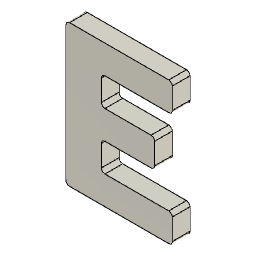
East (Autodesk Fusion 360 design; units mm, degrees)
Autodesk Fusion 360 part; units mm, degrees
sketch "Sketch1" plane through (0, 0, 0) normal (0, 1, 0) x (1, 0, 0)
  line L0 (0, -1.27) -> (0, -49.53)
  line L1 (1.27, -50.8) -> (36.83, -50.8)
  line L2 (38.1, -49.53) -> (38.1, -41.91)
  line L3 (36.83, -40.64) -> (13.97, -40.64)
  line L4 (12.7, -39.37) -> (12.7, -31.75)
  line L5 (13.97, -30.48) -> (30.4855, -30.48)
  line L6 (31.7555, -29.21) -> (31.7555, -21.59)
  line L7 (30.4855, -20.32) -> (13.97, -20.32)
  line L8 (12.7, -19.05) -> (12.7, -11.43)
  line L9 (13.97, -10.16) -> (36.83, -10.16)
  line L10 (38.1, -8.89) -> (38.1, -1.27)
  line L11 (36.83, 0) -> (1.27, 0)
  arc A0 (0, -49.53) -> (1.27, -50.8) centre (1.27, -49.53) ccw
  arc A1 (36.83, -50.8) -> (38.1, -49.53) centre (36.83, -49.53) ccw
  arc A2 (38.1, -41.91) -> (36.83, -40.64) centre (36.83, -41.91) ccw
  arc A3 (12.7, -39.37) -> (13.97, -40.64) centre (13.97, -39.37) ccw
  arc A4 (13.97, -30.48) -> (12.7, -31.75) centre (13.97, -31.75) ccw
  arc A5 (30.4855, -30.48) -> (31.7555, -29.21) centre (30.4855, -29.21) ccw
  arc A6 (31.7555, -21.59) -> (30.4855, -20.32) centre (30.4855, -21.59) ccw
  arc A7 (12.7, -19.05) -> (13.97, -20.32) centre (13.97, -19.05) ccw
  arc A8 (13.97, -10.16) -> (12.7, -11.43) centre (13.97, -11.43) ccw
  arc A9 (36.83, -10.16) -> (38.1, -8.89) centre (36.83, -8.89) ccw
  arc A10 (38.1, -1.27) -> (36.83, 0) centre (36.83, -1.27) ccw
  arc A11 (1.27, 0) -> (0, -1.27) centre (1.27, -1.27) ccw
  point P0 (0, -50.8)
  dimension "d1" = 50.8
  dimension "d2" = 1.27
  constraint vertical L0
  constraint perpendicular L0 L1
  constraint perpendicular L1 L2
  constraint perpendicular L2 L3
  constraint perpendicular L3 L4
  constraint perpendicular L4 L5
  constraint perpendicular L5 L6
  constraint perpendicular L6 L7
  constraint perpendicular L7 L8
  constraint perpendicular L8 L9
  constraint perpendicular L9 L10
  constraint perpendicular L0 L11
  constraint coincident P0 L0
  constraint coincident P0 L1
  constraint tangent L0 A0
  constraint tangent L1 A0
  constraint tangent L1 A1
  constraint tangent L2 A1
  constraint equal A0 A1
  constraint tangent L2 A2
  constraint tangent L3 A2
  constraint equal A0 A2
  constraint tangent L3 A3
  constraint tangent L4 A3
  constraint equal A0 A3
  constraint tangent L4 A4
  constraint tangent L5 A4
  constraint equal A0 A4
  constraint tangent L5 A5
  constraint tangent L6 A5
  constraint equal A0 A5
  constraint tangent L6 A6
  constraint tangent L7 A6
  constraint equal A0 A6
  constraint tangent L7 A7
  constraint tangent L8 A7
  constraint equal A0 A7
  constraint tangent L8 A8
  constraint tangent L9 A8
  constraint equal A0 A8
  constraint tangent L9 A9
  constraint tangent L10 A9
  constraint equal A0 A9
  constraint tangent L10 A10
  constraint tangent L11 A10
  constraint equal A0 A10
  constraint coincident origin L0
  constraint tangent L11 A11
  constraint tangent L0 A11
  constraint equal A0 A11
  measures "d1" distance of origin P0
  measures "d2" radius of A0
extrude "Extrude1" add sketch "Sketch1" along normal blind 6.35
